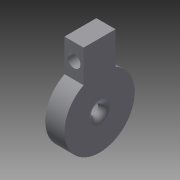
# Autodesk Inventor part: enganche-servo-cable
Saved by Autodesk Inventor 2015 SP1 (Build 190203100, 203)
## iProperties
Created: 2015-07-03
Part Number: enganche-servo-cable
Material: Genérico
Document SubType Name: Modeling
Designer: Javier
Density: 1 g/cm^3
Appearance: Valor por defecto
Author: Javier
Autodesk Inventor part; units mm, degrees
ref_plane "YZ Plane" through (0, 0, 0) normal (1, 0, 0) x (0, 1, 0)
ref_plane "XZ Plane" through (0, 0, 0) normal (0, 1, 0) x (-1, 0, 0)
ref_plane "XY Plane" through (0, 0, 0) normal (0, 0, 1) x (1, 0, 0)
sketch "Boceto1" plane through (0, 0, 0) normal (1, 0, 0) x (0, 1, 0)
  circle A0 centre (0, 0) radius 2.1
  circle A1 centre (0, 0) radius 5.5
  dimension "d0" = 4.2
  dimension "d1" = 11
  constraints: 2 centre point, 2 coincident
  measures "d0" diameter of A0
  measures "d1" diameter of A1
extrude "Extrusión1" add sketch "Boceto1" along normal blind 3
sketch "Boceto2" plane through (3, 0, 0) normal (1, 0, 0) x (0, 0, -1)
  line L0 (0, 0) -> (-10, 0)
  line L1 (-10, 0) -> (-10, 2.5)
  line L2 (-10, 2.5) -> (-3.6594, 2.5)
  line L3 (-3.6594, 2.5) -> (-3.6594, -2.5)
  line L4 (-3.6594, -2.5) -> (-10, -2.5)
  line L5 (-10, -2.5) -> (-10, 0)
  dimension "d4" = 10
  dimension "d5" = 2.5
  dimension "d6" = 5
  constraints: 12 end point, 4 perpendicular, 1 horizontal, 1 vertical
  measures "d4" distance of L0.start L0.end
  measures "d5" distance of L0.end L1.end
  measures "d6" distance of L2.end L3.end
extrude "Extrusión2" add sketch "Boceto2" against normal blind 3
sketch "Boceto3" plane through (3, -2.5, 4.899) normal (0, -1, 0) x (1, 0, 0)
  line L0 (0, 0) -> (-3, 0) projected
  line L1 (0, 0) -> (0, 5.101) projected
  line L2 (0, 5.101) -> (-3, 5.101) projected
  line L3 (-3, 0) -> (-3, 5.101) projected
  circle A0 centre (-1.5, 2.5505) radius 1
  point P0 (-3, -4.899)
  dimension "d19" = 2
  constraints: 1 centre point
  measures "d19" diameter of A0
extrude "Extrusión3" cut sketch "Boceto3" against normal blind 5 contours A0
sketch "Boceto4" plane through (3, 0, 0) normal (1, 0, 0) x (0, 0, -1)
  circle A0 centre (0, 0) radius 2.1 projected
extrude "Extrusión4" add sketch "Boceto4" against normal blind 1
sketch "Boceto5" plane through (3, 0, 0) normal (1, 0, 0) x (0, 0, -1)
  circle A0 centre (0, 0) radius 0.75
  dimension "d15" = 1.5
  constraints: 1 centre point, 1 coincident
  measures "d15" diameter of A0
extrude "Extrusión5" cut sketch "Boceto5" against normal blind 1
fillet "Empalme1" radius 1 1 edges at (3, 0, 0.75)
